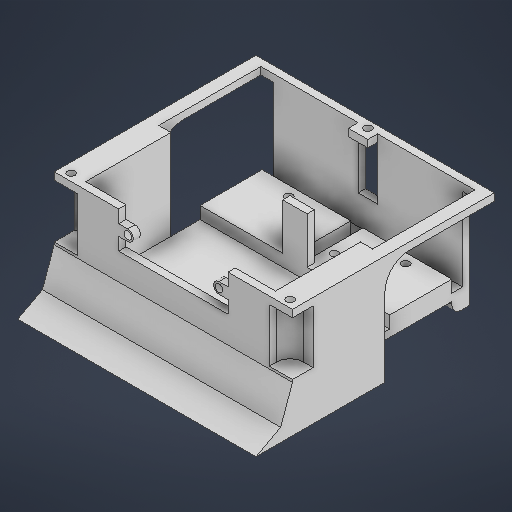
# Autodesk Inventor part: Część1
Saved by Autodesk Inventor 2026 (Build 300175000, 175)
## iProperties
Created: 2026-05-09
Part Number: Część1
Material: Ogólny
Document SubType Name: Modeling
Designer: Patryk Lombardo
Density: 1 g/cm^3
Appearance: Domyślna
Author: Patryk Lombardo
Autodesk Inventor part; units mm, degrees
ref_plane "YZ Plane" through (0, 0, 0) normal (1, 0, 0) x (0, 1, 0)
ref_plane "XZ Plane" through (0, 0, 0) normal (0, 1, 0) x (-1, 0, 0)
ref_plane "XY Plane" through (0, 0, 0) normal (0, 0, 1) x (1, 0, 0)
sketch "Szkic1" plane through (0, 0, 0) normal (0, 1, 0) x (-1, 0, 0)
  line L0 (0, 0) -> (-98, 0)
  line L1 (-98, 0) -> (-98, -98)
  line L2 (-98, -98) -> (0, -98)
  line L3 (0, -98) -> (0, 0)
  line L4 (-88, -98) -> (-88, -53)
  line L5 (-88, -53) -> (-98, -53)
  line L6 (-10, -98) -> (-10, -53)
  line L7 (-10, -53) -> (0, -53)
  dimension "d0" = 98
  dimension "d1" = 98
  dimension "d2" = 45
  dimension "d3" = 10
  dimension "d4" = 10
  constraints: 16 end point, 6 point on line, 3 perpendicular, 2 parallel, 1 horizontal, 1 vertical
  measures "d0" distance of L0.end L1.end
  measures "d1" distance of L1.end L2.end
  measures "d2" distance of L4.start L4.end
  measures "d3" distance of L4.end L5.end
  measures "d4" distance of L6.end L7.end
extrude "Wyciągnięcie proste1" add sketch "Szkic1" along normal blind 8 contours L3 L7 L6 L2 L4 L5 L1 L0
sketch "Szkic2" plane through (0, 8, 0) normal (0, 1, 0) x (1, 0, 0)
  line L0 (0, 0) -> (98, 0)
  line L1 (98, 0) -> (98, 98)
  line L2 (98, 98) -> (0, 98)
  line L3 (0, 98) -> (0, 0)
  line L4 (10, 18) -> (88, 18)
  line L5 (88, 18) -> (88, 65)
  line L6 (88, 65) -> (10, 65)
  line L7 (10, 65) -> (10, 18)
  line L8 (98, 0) -> (98, 18) construction
  line L9 (88, 18) -> (98, 18) construction
  line L10 (98, 15) -> (0, 15)
  line L11 (88, 18) -> (88, 15) construction
  line L12 (98, 15) -> (98, 53)
  line L13 (88, 53) -> (98, 53)
  line L14 (0, 15) -> (0, 53)
  line L15 (10, 53) -> (0, 53)
  line L16 (10, 98) -> (10, 95)
  line L17 (10, 95) -> (88, 95)
  line L18 (88, 95) -> (88, 98)
  line L19 (44, 65) -> (44, 68)
  line L20 (44, 68) -> (54, 68)
  line L21 (54, 68) -> (54, 65)
  dimension "d7" = 98
  dimension "d8" = 98
  dimension "d9" = 47
  dimension "d10" = 78
  dimension "d11" = 18
  dimension "d12" = 10
  dimension "d13" = 3
  dimension "d14" = 38
  dimension "d15" = 38
  dimension "d16" = 3
  dimension "d17" = 78
  dimension "d30" = 3
  dimension "d31" = 10
  dimension "d32" = 44
  dimension "d36" = 10
  dimension "d37" = 0
  dimension "d38" = 38
  constraints: 44 end point, 13 perpendicular, 12 point on line, 4 parallel, 2 horizontal
  measures "d7" distance of L0.end L1.end
  measures "d8" distance of L1.end L2.end
  measures "d9" distance of L4.end L5.end
  measures "d10" distance of L5.end L6.end
  measures "d11" distance of L0.end L8.end
  measures "d12" distance of L4.end L8.end
  measures "d13" distance of L4.end L11.end
  measures "d14" distance of L10.start L12.end
  measures "d15" distance of L14.end L10.end
  measures "d16" distance of L17.end L18.end
  measures "d17" distance of L16.end L17.end
  measures "d30" distance of L19.start L19.end
  measures "d31" distance of L19.end L20.end
  measures "d32" distance between parallel lines of L1 L21
  measures "d36" distance between parallel lines of L18 L1
  measures "d37" distance from line of point (98, 15) L1
  measures "d38" distance from line of point (98, 15) L13
extrude "Wyciągnięcie proste2" add sketch "Szkic2" along normal blind 37 contours L3 L15 L7 L4 L5 L13 L1 L10 | L2 L18 L17 L16
sketch "Szkic3" plane through (0, 45, 0) normal (0, 1, 0) x (1, 0, 0)
  line L0 (0, 0) -> (0, 98)
  line L1 (0, 98) -> (5, 98)
  line L2 (5, 98) -> (10, 98)
  line L3 (10, 98) -> (88, 98)
  line L4 (88, 98) -> (93, 98)
  line L5 (93, 98) -> (98, 98)
  line L6 (5, 98) -> (5, 53)
  line L7 (5, 53) -> (0, 53)
  line L8 (93, 98) -> (93, 53)
  line L9 (93, 53) -> (88, 53)
  line L10 (88, 53) -> (88, 98)
  line L11 (88, 98) -> (88, 95)
  line L12 (88, 95) -> (93, 95)
  line L13 (5, 95) -> (10, 95)
  line L14 (10, 95) -> (10, 98)
  line L15 (93, 53) -> (98, 53)
  line L16 (98, 53) -> (98, 98)
  dimension "d20" = 98
  dimension "d21" = 5
  dimension "d22" = 5
  dimension "d23" = 78
  dimension "d24" = 5
  dimension "d25" = 5
  dimension "d26" = 45
  dimension "d27" = 3
  constraints: 34 end point, 11 point on line, 7 perpendicular, 2 horizontal, 2 vertical
  measures "d20" distance of L0.start L0.end
  measures "d21" distance of L0.end L1.end
  measures "d22" distance of L1.end L2.end
  measures "d23" distance of L2.end L3.end
  measures "d24" distance of L3.end L4.end
  measures "d25" distance of L4.end L5.end
  measures "d26" distance of L4.end L8.end
  measures "d27" distance of L13.end L2.end
extrude "Wyciągnięcie proste3" add sketch "Szkic3" against normal blind 3 contours L4 L8 L12 L10 | L0 L1 L6 L7 | L2 L14 L13 L6 | L5 L16 L15 L8
extrude "Wyciągnięcie proste4" add sketch "Szkic2" along normal blind 24 contours L19 L20 L21 L6
sketch "Szkic4" plane through (98, 0, 0) normal (1, 0, 0) x (0, 0, -1)
  line L0 (0, 0) -> (15, 8)
  line L1 (15, 8) -> (15, 0)
  line L2 (15, 0) -> (0, 0)
  line L3 (15, 8) -> (0, 8)
  line L4 (0, 8) -> (0, 0)
  dimension "d41" = 15
  dimension "d42" = 8
  constraints: 10 end point, 2 perpendicular, 1 horizontal, 1 vertical
  measures "d41" distance of L1.end L0.start
  measures "d42" distance of L0.end L1.end
extrude "Wyciągnięcie proste5" cut sketch "Szkic4" against normal through all contours L4 L3 L0
sketch "Szkic5" plane through (0, 0, 0) normal (0, -1, 0) x (1, 0, 0)
  line L0 (0, 0) -> (0, -13) construction
  line L1 (0, -13) -> (12, -13) construction
  line L2 (12, -13) -> (22, -13)
  line L3 (22, -13) -> (76, -13) construction
  line L4 (76, -13) -> (86, -13)
  line L5 (12, -13) -> (12, -53)
  line L6 (12, -53) -> (22, -53)
  line L7 (22, -53) -> (22, -13)
  line L8 (76, -13) -> (76, -53)
  line L9 (76, -53) -> (86, -53)
  line L10 (86, -53) -> (86, -13)
  line L11 (76, -53) -> (22, -53)
  line L12 (76, -43) -> (22, -43)
  line L13 (44, -53) -> (44, -83)
  line L14 (44, -83) -> (54, -83)
  line L15 (54, -83) -> (54, -53)
  line L16 (54, -73) -> (44, -73)
  point P0 (49, -83)
  dimension "d45" = 13
  dimension "d46" = 12
  dimension "d47" = 10
  dimension "d48" = 10
  dimension "d49" = 54
  dimension "d50" = 40
  dimension "d51" = 10
  dimension "d52" = 30
  dimension "d53" = 10
  dimension "d54" = 22
  dimension "d55" = 10
  constraints: 34 end point, 11 point on line, 8 perpendicular, 3 vertical, 1 horizontal, 1 midpoint, 1 parallel
  measures "d45" distance of L0.start L0.end
  measures "d46" distance of L0.end L1.end
  measures "d47" distance of L1.end L2.end
  measures "d48" distance of L3.end L4.end
  measures "d49" distance of L2.end L3.end
  measures "d50" distance of L1.end L5.end
  measures "d51" distance between parallel lines of L11 L12
  measures "d52" distance of L13.start L13.end
  measures "d53" distance of L13.end L14.end
  measures "d54" distance from line of L6.end L13
  measures "d55" distance from line of point (49, -83) L16
extrude "Wyciągnięcie proste6" cut sketch "Szkic5" against normal blind 3.5 contours L2 L7 L6 L5 | L12 L8 L11 L7 | L8 L4 L10 L9 | L11 L15 L16 L13
extrude "Wyciągnięcie proste7" cut sketch "Szkic5" against normal through all contours L16 L15 L14 L13
sketch "Szkic6" plane through (0, 0, 0) normal (0, -1, 0) x (1, 0, 0)
  line L0 (0, 0) -> (0, -53) construction
  line L1 (0, -53) -> (0, -98) construction
  line L2 (0, -53) -> (10, -53) construction
  line L3 (10, -53) -> (10, -75.5) construction
  line L4 (10, -60.5) -> (10, -90.5)
  line L5 (10, -60.5) -> (46.5, -60.5)
  line L6 (46.5, -60.5) -> (46.5, -90.5)
  line L7 (46.5, -90.5) -> (10, -90.5)
  line L8 (46.5, -90.5) -> (51.5, -90.5) construction
  line L9 (51.5, -90.5) -> (88, -90.5)
  line L10 (88, -90.5) -> (88, -60.5)
  line L11 (88, -60.5) -> (51.5, -60.5)
  line L12 (51.5, -60.5) -> (51.5, -90.5)
  line L13 (10, -75.5) -> (25, -75.5) construction
  line L14 (25, -64.5) -> (25, -86.5) construction
  circle A0 centre (25, -86.5) radius 1.6
  line L15 (88, -75.5) -> (73, -75.5) construction
  line L16 (73, -64.5) -> (73, -86.5) construction
  circle A1 centre (73, -86.5) radius 1.6
  line L17 (25, -75.5) -> (43.25, -75.5) construction
  circle A2 centre (43.25, -75.5) radius 1.6
  line L18 (73, -75.5) -> (54.75, -75.5) construction
  circle A3 centre (54.75, -75.5) radius 1.6
  line L19 (51.5, -60.5) -> (46.5, -60.5)
  line L20 (51.5, -82.5) -> (46.5, -82.5)
  point P0 (80.5, -75.5)
  point P1 (49, -82.5)
  dimension "d60" = 53
  dimension "d61" = 45
  dimension "d62" = 10
  dimension "d63" = 22.5
  dimension "d64" = 30
  dimension "d65" = 36.5
  dimension "d66" = 5
  dimension "d67" = 36.5
  dimension "d68" = 30
  dimension "d73" = 22
  dimension "d74" = 15
  dimension "d75" = 15
  dimension "d76" = 3.2
  dimension "d78" = 15
  dimension "d79" = 22
  dimension "d80" = 15
  dimension "d81" = 3.2
  dimension "d85" = 18.25
  dimension "d86" = 3.2
  dimension "d87" = 18.25
  dimension "d88" = 3.2
  dimension "d89" = 22
  constraints: 42 end point, 9 perpendicular, 7 midpoint, 5 horizontal, 4 centre point, 4 coincident, 4 point on line, 4 vertical
  measures "d60" distance of L0.start L0.end
  measures "d61" distance of L0.end L1.end
  measures "d62" distance of L0.end L2.end
  measures "d63" distance of L2.end L3.end
  measures "d64" distance of L4.start L4.end
  measures "d65" distance of L6.end L4.end
  measures "d66" distance of L6.end L8.end
  measures "d67" distance of L8.end L9.end
  measures "d68" distance of L11.end L8.end
  measures "d73" distance of L14.start L14.end
  measures "d74" distance of L13.start L13.end
  measures "d75" distance between parallel lines of L5 L13
  measures "d76" diameter of A0
  measures "d78" distance of L15.start L15.end
  measures "d79" distance of L16.start L16.end
  measures "d80" distance from line of point (80.5, -75.5) L9
  measures "d81" diameter of A1
  measures "d85" distance of L13.end L17.end
  measures "d86" diameter of A2
  measures "d87" distance of L15.end L18.end
  measures "d88" diameter of A3
  measures "d89" distance from line of point (49, -82.5) L19
extrude "Wyciągnięcie proste8" add sketch "Szkic6" against normal blind 13 contours L5 L6 L7 L4 | L11 L10 L9 L12 | A0 | A1 | A2 | A3
extrude "Wyciągnięcie proste9" cut sketch "Szkic6" against normal blind 5 contours L5 L6 L7 L4 | L19 L12 L20 L6 | L11 L10 L9 L12 | A0 | A1 | A2 | A3
extrude "Wyciągnięcie proste10" cut sketch "Szkic6" against normal through all contours A0 | A1 | A2 | A3
fillet "Zaokrąglenie1" radius 4 3 edges at (49, 0, -83) (69.75, 0, -90.5) (28.25, 0, -90.5)
fillet "Zaokrąglenie2" radius 10 2 edges at (95.5, 42, -53) (2.5, 42, -53)
sketch "Szkic7" plane through (0, 13, 0) normal (0, 1, 0) x (1, 0, 0)
  line L0 (0, 0) -> (0, 60.5) construction
  line L1 (0, 60.5) -> (10, 60.5) construction
  line L2 (10, 60.5) -> (10, 65)
  line L3 (10, 65) -> (88, 65)
  line L4 (88, 65) -> (88, 60.5)
  line L5 (88, 60.5) -> (10, 60.5)
  dimension "d92" = 10
  dimension "d93" = 60.5
  dimension "d94" = 4.5
  dimension "d95" = 78
  constraints: 12 end point, 4 perpendicular, 2 vertical
  measures "d92" distance of L0.end L1.end
  measures "d93" distance of L0.start L0.end
  measures "d94" distance of L3.end L4.end
  measures "d95" distance of L2.end L3.end
extrude "Wyciągnięcie proste11" cut sketch "Szkic7" against normal blind 5
sketch "Szkic8" plane through (0, 45, 0) normal (0, 1, 0) x (1, 0, 0)
  line L0 (0, 0) -> (0, 15) construction
  line L1 (0, 15) -> (0, 18)
  line L2 (0, 18) -> (4, 18)
  circle A0 centre (4, 18) radius 1.6
  circle A1 centre (4, 18) radius 5.5
  line L3 (9.5, 18) -> (9.5, 10)
  line L4 (4, 23.5) -> (-4, 23.5)
  line L5 (-4, 23.5) -> (-4, 10)
  line L6 (-4, 10) -> (9.5, 10)
  line L7 (0, 15) -> (98, 15) construction
  line L8 (98, 15) -> (98, 18) construction
  line L9 (98, 18) -> (94, 18) construction
  circle A2 centre (94, 18) radius 1.6
  circle A3 centre (94, 18) radius 5.5
  line L10 (94, 23.5) -> (102, 23.5)
  line L11 (102, 23.5) -> (102, 10)
  line L12 (102, 10) -> (88.5, 10)
  line L13 (88.5, 10) -> (88.5, 18)
  line L14 (98, 21.7749) -> (98, 15)
  line L15 (98, 15) -> (89.3902, 15)
  line L16 (98, 21.7749) -> (98, 23.5)
  line L17 (89.3902, 15) -> (88.5, 15)
  line L18 (9.5, 15) -> (8.6098, 15)
  line L19 (0, 15) -> (8.6098, 15)
  line L20 (0, 15) -> (0, 21.7749)
  line L21 (0, 23.5) -> (0, 21.7749)
  dimension "d98" = 15
  dimension "d99" = 4
  dimension "d100" = 3
  dimension "d101" = 3.2
  dimension "d102" = 11
  dimension "d103" = 8
  dimension "d104" = 8
  dimension "d105" = 98
  dimension "d106" = 3
  dimension "d107" = 4
  dimension "d108" = 11
  dimension "d109" = 3.2
  dimension "d110" = 8
  dimension "d111" = 8
  constraints: 44 end point, 8 point on circle, 7 point on line, 6 perpendicular, 4 centre point, 4 coincident, 4 tangent, 4 vertical, 3 horizontal, 2 collinear, 2 midpoint, 1 parallel
  measures "d98" distance of L0.start L0.end
  measures "d99" distance of L1.end L2.end
  measures "d100" distance of L0.end L1.end
  measures "d101" diameter of A0
  measures "d102" diameter of A1
  measures "d103" distance of L3.start L3.end
  measures "d104" distance of L4.start L4.end
  measures "d105" distance of L0.end L7.end
  measures "d106" distance of L7.end L8.end
  measures "d107" distance of L8.end L9.end
  measures "d108" diameter of A3
  measures "d109" diameter of A2
  measures "d110" distance of L10.start L10.end
  measures "d111" distance of L12.end L13.end
extrude "Wyciągnięcie proste12" cut sketch "Szkic8" against normal blind 25 contours L19 A1 L20 L1 | A0 | L1 L20 A1 L19 | L18 L3 L6 L5 L4 L21 A1 | A1 L3 L18 | L21 L4 A1 | A2 | A3 L15 L14 | A3 L16 L10 L11 L12 L13 L17 | L14 L15 A3 | A3 L10 L16 | L17 L13 A3
extrude "Wyciągnięcie proste13" add sketch "Szkic8" against normal blind 3 contours L1 L20 A1 L19 | A1 L3 L18 | L21 L4 A1 | L14 L15 A3 | A3 L10 L16 | L17 L13 A3 picked at (4.2676, 15.4706) picked at (97.2, 18.2583)
sketch "Szkic9" plane through (0, 45, 0) normal (0, 1, 0) x (1, 0, 0)
  line L0 (0, 0) -> (0, 98) construction
  line L1 (0, 98) -> (49, 98) construction
  line L2 (49, 98) -> (49, 95) construction
  line L3 (49, 95) -> (49, 91) construction
  circle A0 centre (49, 95) radius 1.6
  line L4 (45, 91) -> (53, 91)
  line L5 (45, 91) -> (45, 98)
  line L6 (53, 91) -> (53, 98)
  line L7 (53, 98) -> (45, 98)
  dimension "d116" = 3
  dimension "d117" = 4
  dimension "d118" = 49
  dimension "d119" = 98
  dimension "d120" = 3.2
  dimension "d121" = 8
  constraints: 16 end point, 4 perpendicular, 2 coincident, 2 point on line, 2 vertical, 1 centre point, 1 horizontal, 1 midpoint
  measures "d116" distance of L1.end L2.end
  measures "d117" distance of L2.end L3.end
  measures "d118" distance of L0.end L1.end
  measures "d119" distance of L0.start L0.end
  measures "d120" diameter of A0
  measures "d121" distance of L4.start L4.end
extrude "Wyciągnięcie proste14" cut sketch "Szkic9" against normal blind 25 contours A0 | L5 L7 L6 L4
extrude "Wyciągnięcie proste15" add sketch "Szkic9" against normal blind 3
sketch "Szkic10" plane through (98, 45, -15) normal (1, 0, 0) x (0, 0, -1)
  line L0 (-15, -45) -> (-5, -45) construction
  line L1 (-5, -45) -> (-5, -40) construction
  line L2 (-5, -40) -> (0, -40)
  line L3 (0, -40) -> (0, -26)
  line L4 (-5, -40) -> (0, -26)
  dimension "d126" = 10
  dimension "d128" = 5
  dimension "d129" = 5
  dimension "d130" = 14
  constraints: 10 end point, 2 perpendicular, 1 horizontal, 1 vertical
  measures "d126" distance of L0.start L0.end
  measures "d128" distance of L0.end L1.end
  measures "d129" distance of L1.end L2.end
  measures "d130" distance of L2.end L3.end
extrude "Wyciągnięcie proste16" add sketch "Szkic10" against normal blind 98
sketch "Szkic11" plane through (0, 45, -15) normal (0, 0, 1) x (1, 0, 0)
  line L0 (0, -45) -> (49, -45) construction
  line L1 (49, -45) -> (49, -15) construction
  line L2 (26.5, -15) -> (71.5, -15)
  line L3 (26.5, -15) -> (26.5, 0)
  line L4 (26.5, 0) -> (71.5, 0)
  line L5 (71.5, 0) -> (71.5, -15)
  line L6 (49, -15) -> (49, -7.5) construction
  line L7 (30.25, -7.5) -> (67.75, -7.5) construction
  circle A0 centre (67.75, -7.5) radius 1.6
  circle A1 centre (30.25, -7.5) radius 1.6
  circle A2 centre (67.75, -7.5) radius 2.25
  circle A3 centre (30.25, -7.5) radius 2.25
  line L8 (30.25, -5.25) -> (26.5, -5.25)
  line L9 (30.25, -9.75) -> (26.5, -9.75)
  line L10 (67.75, -9.75) -> (71.5, -9.75)
  line L11 (67.75, -5.25) -> (71.5, -5.25)
  point P0 (0, -45)
  dimension "d133" = 30
  dimension "d134" = 49
  dimension "d135" = 45
  dimension "d136" = 15
  dimension "d137" = 7.5
  dimension "d138" = 37.5
  dimension "d139" = 3.2
  dimension "d140" = 3.2
  dimension "d141" = 4.5
  dimension "d142" = 4.5
  constraints: 24 end point, 8 point on line, 5 coincident, 5 perpendicular, 4 centre point, 4 point on circle, 3 horizontal, 2 midpoint, 2 tangent, 2 vertical
  measures "d133" distance of L0.end L1.end
  measures "d134" distance of L0.start L0.end
  measures "d135" distance of L3.end L4.end
  measures "d136" distance of L4.end L2.end
  measures "d137" distance of L1.end L6.end
  measures "d138" distance of L7.start L7.end
  measures "d139" diameter of A1
  measures "d140" diameter of A0
  measures "d141" diameter of A2
  measures "d142" diameter of A3
extrude "Wyciągnięcie proste17" cut sketch "Szkic11" against normal blind 11 contours L3 L9 A3 L8 L4 L5 L11 A2 L10 L2 | A0 | A1
equation "\"d12\" = -0.5 * d10 + 0.5 * d8"
equation "\"d15\" = d14"
equation "\"d48\" = d47"
equation "\"d63\" = 0.5 * d61"
equation "\"d67\" = d65"
equation "\"d68\" = d64"
equation "\"d87\" = d85"
